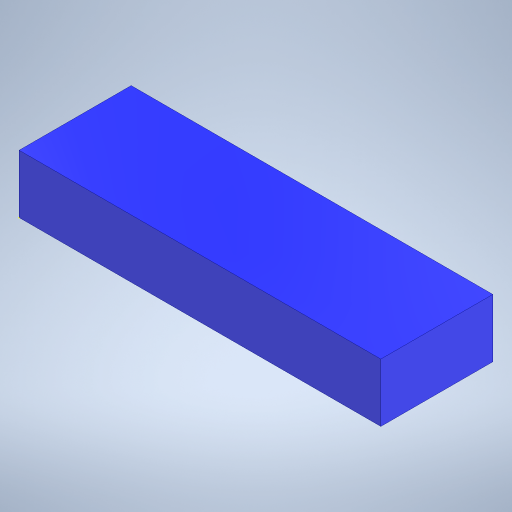
# Autodesk Inventor part: battery_12
Saved by Autodesk Inventor 2023 (Build 270158000, 158)
## iProperties
Created: 2022-12-19
Part Number: battery_12
Material: Generic
Document SubType Name: Modeling
Designer: LAB-505
Density: 1.7043 g/cm^3
Appearance: Blue - Wall Paint - Glossy
Mass: 317 g
Surface Area: 250.3 cm^2
Volume: 186 cm^3
Author: LAB-505
Autodesk Inventor part; units mm, degrees
ref_plane "YZ Plane" through (0, 0, 0) normal (1, 0, 0) x (0, 1, 0)
ref_plane "XZ Plane" through (0, 0, 0) normal (0, 1, 0) x (-1, 0, 0)
ref_plane "XY Plane" through (0, 0, 0) normal (0, 0, 1) x (1, 0, 0)
sketch "Sketch1" plane through (0, 0, 0) normal (1, 0, 0) x (0, 1, 0)
  point P0 (0, 0)
sketch "Sketch2" plane through (0, 0, 0) normal (1, 0, 0) x (0, 1, 0)
  line L0 (0, 0) -> (25, 0)
  line L1 (25, 0) -> (25, -48)
  line L2 (25, -48) -> (0, -48)
  line L3 (0, -48) -> (0, 0)
  dimension "d0" = 25
  dimension "d1" = 48
  constraints: 8 end point, 2 parallel, 1 horizontal, 1 perpendicular
  measures "d0" distance of L1.end L2.end
  measures "d1" distance of L0.end L1.end
extrude "Extrusion1" add sketch "Sketch2" along normal blind 155
body "Solid1"
